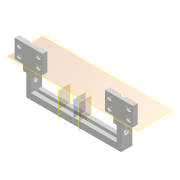
# Autodesk Inventor part: frontChassis_final
Saved by Autodesk Inventor 2018 (Build 220112000, 112)
## iProperties
Created: 2017-10-21
Part Number: frontChassis_final
Material: Generic
Document SubType Name: Modeling
Designer: Prakash
Density: 1 g/cm^3
Appearance: Default
d0: 1.500 mm
d1: 10.000 mm
d2: 18.000 mm
d3: 18.000 mm
d4: 30.000 mm
d5: 0.00 deg
d8: 10.000 mm
d9: 0.00 deg
d10: 3.588 mm
d11: 3.588 mm
d12: 34.763 mm
d13: 0.00 deg
d15: 9.763 mm
d16: 9.525 mm
d17: 8.000 mm
d19: 0.00 deg
d20: 4.000 mm
d21: 0.00 deg
d22: 10.000 mm
d25: 10.000 mm
d26: 5.000 mm
d27: 70.000 mm
d28: 0.00 deg
d74: 7.000 mm
d75: 7.000 mm
d76: 7.500 mm
d77: 7.500 mm
d79: 7.500 mm
d80: 7.500 mm
d81: 3.000 mm
d89: 8.000 mm
d90: 3.175 mm
d91: 0.00 deg
d104: -68.000 mm
d117: 45.250 mm
Author: Prakash
Autodesk Inventor part; units mm, degrees
ref_plane "YZ Plane" through (0, 0, 0) normal (1, 0, 0) x (0, 1, 0)
ref_plane "XZ Plane" through (0, 0, 0) normal (0, 1, 0) x (-1, 0, 0)
ref_plane "XY Plane" through (0, 0, 0) normal (0, 0, 1) x (1, 0, 0)
sketch "Sketch1" plane through (0, 0, 0) normal (0, 0, 1) x (1, 0, 0)
  line L0 (0, 0) -> (45.5394, 0)
  line L1 (45.5394, 0) -> (45.5394, 7.5)
  line L2 (45.5394, 7.5) -> (27.5394, 7.5)
  line L3 (0, 7.5) -> (0, 0)
  line L4 (22.7697, 7.5) -> (22.7697, 9) construction
  arc A0 (18, 7.5) -> (27.5394, 7.5) centre (22.7697, 9) ccw
  circle A1 centre (22.7697, 9) radius 9 construction
  line L5 (18, 7.5) -> (0, 7.5)
  line L6 (27.5394, 7.5) -> (22.7697, 7.5) construction
  line L7 (22.7697, 7.5) -> (18, 7.5) construction
  dimension "d0" = 1.5
  dimension "d1" = 10
  dimension "d2" = 18
  dimension "d3" = 18
  constraints: 16 end point, 5 parallel, 2 centre point, 2 coincident, 2 point on circle, 1 collinear, 1 horizontal, 1 perpendicular, 1 tangent, 1 vertical
  measures "d0" distance of L4.start L4.end
  measures "d1" diameter of A0
  measures "d2" distance of L1.end L2.end
  measures "d3" diameter of A1
extrude "Extrusion1" add sketch "Sketch1" along normal blind 30
sketch "Sketch3" plane through (0, 0, 0) normal (0, 0, -1) x (-1, 0, 0)
  circle A0 centre (-22.7697, 9) radius 9 construction
  arc A1 (-27.5394, 7.5) -> (-18, 7.5) centre (-22.7697, 9) ccw projected
  arc A2 (-27.5394, 7.5) -> (-18, 7.5) centre (-22.7697, 9) ccw projected
  arc A3 (-27.5394, 7.5) -> (-18, 7.5) centre (-22.7697, 9) ccw projected
  circle A4 centre (-22.7697, 9) radius 5
  line L0 (-31.7697, 9) -> (-31.7697, 0)
  line L1 (-13.7697, 9) -> (-13.7697, 0)
  arc A5 (-22.7697, 0) -> (-13.7697, 9) centre (-22.7697, 9) ccw
  line L2 (0, 0) -> (-45.5394, 0) projected
  line L3 (-31.7697, 0) -> (-22.7697, 0)
  line L4 (-22.7697, 0) -> (-13.7697, 0)
  arc A6 (-31.7697, 9) -> (-22.7697, 0) centre (-22.7697, 9) ccw
  arc A7 (-13.7697, 9) -> (-31.7697, 9) centre (-22.7697, 9) ccw
  constraints: 8 end point, 8 point on circle, 3 centre point, 2 coincident, 2 collinear, 2 point on line, 2 tangent, 2 vertical, 1 concentric, 3 other
extrude "Extrusion2" add sketch "Sketch3" along normal blind 10
sketch "Sketch5" plane through (0, 0, -10) normal (0, 0, -1) x (-1, 0, 0)
  line L0 (-31.7697, 0) -> (-13.7697, 0) projected
  line L1 (-22.7697, 0) -> (-19.1822, 0)
  line L2 (-22.7697, 0) -> (-26.3572, 0)
  line L3 (-26.3572, 0) -> (-19.1822, 0)
  line L4 (-19.1822, 0) -> (-19.1822, 18)
  line L5 (-19.1822, 18) -> (-26.3572, 18)
  line L6 (-26.3572, 18) -> (-26.3572, 0)
  arc A0 (-13.7697, 9) -> (-31.7697, 9) centre (-22.7697, 9) ccw projected
  point P0 (0, 0)
  dimension "d10" = 3.5875
  dimension "d11" = 3.5875
  constraints: 12 end point, 2 parallel, 2 point on line, 1 horizontal, 1 midpoint, 1 perpendicular, 1 tangent
  measures "d10" distance of L1.start L1.end
  measures "d11" distance of L1.start L2.end
extrude "Extrusion3" add sketch "Sketch5" along normal blind 34.763
sketch "Sketch6" plane through (26.3572, 5.5172, -10) normal (1, 0, 0) x (0, 0, -1)
  line L0 (-10, 3.4828) -> (0, 3.4828) projected
  line L1 (0, 3.4828) -> (9.763, 3.4828) construction
  circle A0 centre (9.763, 3.4828) radius 4.7625
  circle A1 centre (9.763, 3.4828) radius 4
  point P0 (-10, -5.5172)
  dimension "d15" = 9.763
  dimension "d16" = 9.525
  dimension "d17" = 8
  constraints: 2 centre point, 2 coincident, 2 end point, 1 horizontal
  measures "d15" distance of L0.end L1.end
  measures "d16" diameter of A0
  measures "d17" diameter of A1
extrude "Extrusion4" cut sketch "Sketch6" against normal up to next contours A0 | A1
sketch "Sketch7" plane through (19.1822, 5.5172, -10) normal (-1, 0, 0) x (0, 0, 1)
  circle A0 centre (-9.763, 3.4828) radius 4 projected
  circle A1 centre (-9.763, 3.4828) radius 4.7625 projected
  point P0 (10, -5.5172)
extrude "Extrusion5" add sketch "Sketch7" against normal blind 4
sketch "Sketch8" plane through (19.1822, 5.5172, -10) normal (-1, 0, 0) x (0, 0, 1)
  line L0 (-34.763, -5.5172) -> (-34.763, 12.4828) projected
  line L1 (-34.763, 12.4828) -> (-24.763, 12.4828)
  line L2 (-24.763, 12.4828) -> (-24.763, 5.9828)
  line L3 (-24.763, 5.9828) -> (-34.763, 5.9828)
  line L4 (-34.763, 5.9828) -> (-34.763, 12.4828)
  line L5 (-34.763, -5.5172) -> (-24.763, -5.5172)
  line L6 (-24.763, -5.5172) -> (-24.763, 0.9828)
  line L7 (-24.763, 0.9828) -> (-34.763, 0.9828)
  line L8 (-34.763, 0.9828) -> (-34.763, -5.5172)
  point P0 (10, -5.5172)
  dimension "d22" = 10
  dimension "d25" = 10
  dimension "d26" = 5
  constraints: 16 end point, 4 parallel, 2 horizontal, 2 perpendicular, 1 collinear
  measures "d22" distance of L2.end L3.end
  measures "d25" distance of L6.end L7.end
  measures "d26" distance between parallel lines of L7 L3
extrude "Extrusion6" add sketch "Sketch8" along normal blind 70
sketch "Sketch11" plane through (0, 7.5, 30) normal (0, 1, 0) x (1, 0, 0)
  line L0 (13.7697, 30) -> (0, 30) projected
  line L1 (7, 30) -> (7, 0)
  line L2 (18, 0) -> (0, 0) projected
  line L3 (38.5394, 30) -> (38.5394, 0)
  line L4 (0, 30) -> (0, 0) projected
  line L5 (45.5394, 30) -> (45.5394, 0) projected
  line L6 (45.5394, 30) -> (31.7697, 30) projected
  line L7 (45.5394, 0) -> (27.5394, 0) projected
  point P0 (7, 22.5)
  point P1 (7, 7.5)
  point P2 (38.5394, 22.5)
  point P3 (38.5394, 7.5)
  dimension "d74" = 7
  dimension "d75" = 7
  dimension "d76" = 7.5
  dimension "d77" = 7.5
  dimension "d79" = 7.5
  dimension "d80" = 7.5
  constraints: 8 point on line, 4 end point, 2 vertical
  measures "d74" distance between parallel lines of L4 L1
  measures "d75" distance between parallel lines of L5 L3
  measures "d76" distance of L1.start point (7, 22.5)
  measures "d77" distance of L1.end point (7, 7.5)
  measures "d79" distance of L3.start point (38.539, 22.5)
  measures "d80" distance of L3.end point (38.539, 7.5)
hole "Hole3" at (7, 7.5, 7.5) at (7, 7.5, 22.5) at (38.5394, 7.5, 7.5) at (38.5394, 7.5, 22.5) direction (0, -1, 0) diameter 3 end up to face face through (19.7697, 0, 20) facing (0, -1, 0)
sketch "Sketch13" plane through (0, 0, 30) normal (0, -1, 0) x (1, 0, 0)
  circle A0 centre (7, -7.5) radius 1.5 projected
  circle A1 centre (38.5394, -7.5) radius 1.5 projected
  circle A2 centre (38.5394, -22.5) radius 1.5 projected
  circle A3 centre (7, -22.5) radius 1.5 projected
  line L0 (11, -9.8094) -> (7, -12.1188)
  line L1 (7, -12.1188) -> (3, -9.8094)
  line L2 (3, -9.8094) -> (3, -5.1906)
  line L3 (3, -5.1906) -> (7, -2.8812)
  line L4 (7, -2.8812) -> (11, -5.1906)
  line L5 (11, -5.1906) -> (11, -9.8094)
  line L6 (11, -20.1906) -> (11, -24.8094)
  line L7 (11, -24.8094) -> (7, -27.1188)
  line L8 (7, -27.1188) -> (3, -24.8094)
  line L9 (3, -24.8094) -> (3, -20.1906)
  line L10 (3, -20.1906) -> (7, -17.8812)
  line L11 (7, -17.8812) -> (11, -20.1906)
  line L12 (42.5394, -20.1906) -> (42.5394, -24.8094)
  line L13 (42.5394, -24.8094) -> (38.5394, -27.1188)
  line L14 (38.5394, -27.1188) -> (34.5394, -24.8094)
  line L15 (34.5394, -24.8094) -> (34.5394, -20.1906)
  line L16 (34.5394, -20.1906) -> (38.5394, -17.8812)
  line L17 (38.5394, -17.8812) -> (42.5394, -20.1906)
  line L18 (38.5394, -2.8812) -> (42.5394, -5.1906)
  line L19 (42.5394, -5.1906) -> (42.5394, -9.8094)
  line L20 (42.5394, -9.8094) -> (38.5394, -12.1188)
  line L21 (38.5394, -12.1188) -> (34.5394, -9.8094)
  line L22 (34.5394, -9.8094) -> (34.5394, -5.1906)
  line L23 (34.5394, -5.1906) -> (38.5394, -2.8812)
  line L24 (0, -30) -> (0, 0) projected
  line L25 (45.5394, -30) -> (45.5394, 0) projected
  point P0 (38.5394, -22.5)
  point P1 (38.5394, -7.5)
  dimension "d89" = 8
  constraints: 48 end point, 4 coincident, 4 parallel, 3 equal length, 52 other
  measures "d89" distance between parallel lines of L0 L3
extrude "Extrusion7" cut sketch "Sketch13" against normal blind 3.175
mirror "Mirror1" about plane through (-50.8178, 14.75, -39.763) normal (-1, 0, 0) of "Extrusion6", "Extrusion3", "Extrusion5", "Extrusion4", "Extrusion2", "Extrusion1", "Hole3", "Extrusion7"
ref_plane "Work Plane1" through (-41.6428, 5.5172, -10) normal (1, 0, 0) x (0, 0, -1)
ref_plane "Work Plane2" through (-75.5678, 5.5172, -10) normal (1, 0, 0) x (0, 0, -1)
ref_plane "Work Plane4" through (-133.4053, 9, 0) normal (0, 0, 1) x (1, 0, 0)
split body "Split1" result two bodies by plane through (-133.4053, 9, 0) normal (0, 0, 1) first body at (-120.4821, 0.5, 13.2698) (18.8465, 0.5, 16.7302)
ref_plane "Halfway plane" through (-50.8178, 5.5172, -10) normal (-1, 0, 0) x (0, 0, 1)
body "Solid2"
body "Solid3"
